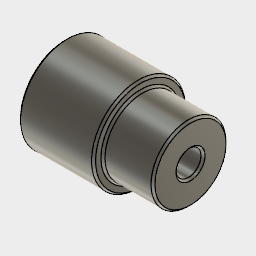
Part A (Autodesk Fusion 360 design; units mm, degrees)
Autodesk Fusion 360 part; units mm, degrees
sketch "Sketch1" plane through (0, 0, 0) normal (0, 0, 1) x (1, 0, 0)
  line L0 (0, 0) -> (0, 11.9062)
  line L1 (0, 11.9062) -> (19.05, 11.9063)
  line L2 (19.05, 11.9063) -> (19.05, 9.525)
  line L3 (19.05, 9.525) -> (31.75, 9.525)
  line L4 (31.75, 9.525) -> (31.75, 0)
  line L5 (31.75, 0) -> (0, 0)
  dimension "d1" = 11.9062
  dimension "d2" = 9.525
  dimension "d3" = 12.7
  dimension "d4" = 19.05
  measures "d1" distance of L0.start L0.end
  measures "d2" distance of L3 L5
  measures "d3" distance of L2.end L3.end
  measures "d4" distance of L0.end L1.end
revolve "Revolve1" add sketch "Sketch1" angle 360 about axis through (31.75, 0, 0) along (-1, 0, 0)
hole "Hole1" at (31.75, 0, 0) direction (-1, 0, 0) diameter 6.35 depth 19.05 tip angle 118
chamfer "Chamfer1" distance 0.508 angle 45 5 edges at (0, -4.3055, 11.1005) (19.05, -4.3055, 11.1005) (19.05, -3.4444, 8.8804) (31.75, -3.4444, 8.8804) (31.75, -2.9601, 1.1481)
equation "d1 = ( 15 / 32 ) * 1 in"
